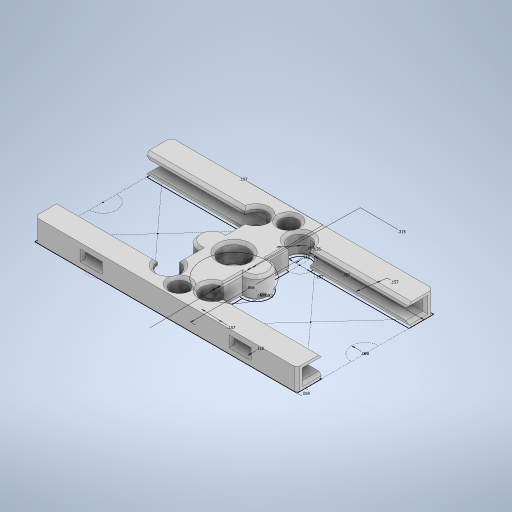
# Autodesk Inventor part: DualSensorClip-v2
Saved by Autodesk Inventor 2023 (Build 270158030, 158C)
## iProperties
Created: 2024-03-05
Part Number: DualSensorClip-v2
Material: Generic
Document SubType Name: Modeling
Designer: lvrectanus0
Density: 1 g/cm^3
Appearance: Default
Author: lvrectanus0
Autodesk Inventor part; units mm, degrees
ref_plane "YZ Plane" through (0, 0, 0) normal (1, 0, 0) x (0, 1, 0)
ref_plane "XZ Plane" through (0, 0, 0) normal (0, 1, 0) x (-1, 0, 0)
ref_plane "XY Plane" through (0, 0, 0) normal (0, 0, 1) x (1, 0, 0)
sketch "Sketch1" plane through (0, 0, 0) normal (0, 1, 0) x (-1, 0, 0)
  circle A0 centre (0, 0) radius 2.5
  circle A1 centre (0, 0) radius 4
  arc A2 (-3.21875, 2.374794) -> (-3.21875, -2.374794) centre (-4, 0) ccw
  line L0 (-24, 11) -> (-4, 11) construction
  line L1 (-4, 11) -> (-4, -11) construction
  line L2 (-4, -11) -> (-24, -11) construction
  line L3 (-24, -11) -> (-24, 11) construction
  line L4 (-24, 11) -> (-4, -11) construction
  line L5 (-4, 11) -> (-24, -11) construction
  arc A3 (-24, -2.5) -> (-24, 2.5) centre (-24, 0) ccw construction
  line L6 (-4, -8) -> (-24, -8) construction
  line L7 (-4, 8) -> (-24, 8) construction
  line L8 (-24, -11) -> (-3.228757, -11) construction
  line L9 (-3.228757, -11) -> (-3.228757, -12.5) construction
  line L10 (-3.228757, -12.5) -> (-24, -12.5)
  line L11 (-24, -12.5) -> (-24, -11)
  line L12 (-4, 11) -> (-24, 11) construction
  line L13 (-24, 11) -> (-24, 12.5)
  line L14 (-24, 12.5) -> (-4, 12.5)
  line L15 (-4, 12.5) -> (-4, 11) construction
  line L16 (-24, 8) -> (-24, 11)
  line L17 (-24, -8) -> (-24, -11)
  circle A4 centre (-4, -8) radius 2 construction
  circle A5 centre (-4, 8) radius 2 construction
  line L18 (-4, 2.5) -> (-4, 6)
  line L19 (-4, -2.5) -> (-4, -6)
  line L20 (-6, -8) -> (-24, -8)
  line L21 (-24, 8) -> (-6, 8)
  circle A6 centre (-13.614378, -11) radius 2 construction
  arc A7 (-6, -8) -> (-4, -6) centre (-4, -8) ccw
  circle A8 centre (0, -10) radius 1.6
  line L22 (-4, -10) -> (-1.6, -10) construction
  line L23 (0, -4) -> (0, -8.4) construction
  arc A9 (-4, 6) -> (-6, 8) centre (-4, 8) ccw
  arc A10 (3.21875, -2.374794) -> (3.21875, 2.374794) centre (4, 0) ccw
  line L24 (4, 2.5) -> (4, 6)
  line L25 (4, -11) -> (4, 11) construction
  circle A11 centre (13.614378, 11) radius 2 construction
  line L26 (24, -12.5) -> (4, -12.5)
  line L27 (24, -8) -> (6, -8)
  line L28 (4, -8) -> (24, -8) construction
  line L29 (4, -11) -> (24, -11) construction
  line L30 (24, -11) -> (4, -11) construction
  arc A12 (24, 2.5) -> (24, -2.5) centre (24, 0) ccw construction
  line L31 (6, 8) -> (24, 8)
  line L32 (4, 8) -> (24, 8) construction
  line L33 (3.228757, 12.5) -> (24, 12.5)
  line L34 (24, 8) -> (24, 11)
  line L35 (24, 11) -> (3.228757, 11) construction
  line L36 (4, 11) -> (24, 11) construction
  line L37 (4, -11) -> (24, 11) construction
  line L38 (24, 11) -> (24, -11) construction
  line L39 (24, -11) -> (4, 11) construction
  line L40 (4, -2.5) -> (4, -6)
  line L41 (24, 12.5) -> (24, 11)
  line L42 (3.228757, 11) -> (3.228757, 12.5) construction
  line L43 (24, -8) -> (24, -11)
  line L44 (24, -11) -> (24, -12.5)
  circle A13 centre (4, -8) radius 2 construction
  arc A14 (4, -6) -> (6, -8) centre (4, -8) ccw
  line L45 (4, -12.5) -> (4, -11) construction
  arc A15 (6, 8) -> (4, 6) centre (4, 8) ccw
  circle A16 centre (4, 8) radius 2 construction
  line L46 (0, 4) -> (0, 8.4) construction
  line L47 (4, 10) -> (1.6, 10) construction
  circle A17 centre (0, 10) radius 1.6
  line L48 (4, -12.5) -> (-3.228757, -12.5)
  line L49 (3.228757, 12.5) -> (-4, 12.5)
  point P0 (-14, 0)
  point P1 (14, 0)
  dimension "d0" = 5
  dimension "d1" = 8
  dimension "d2" = 2.5
  dimension "d3" = 22
  dimension "d4" = 20
  dimension "d5" = 2.5
  dimension "d6" = 3
  dimension "d7" = 3
  dimension "d8" = 1.5
  dimension "d9" = 1.5
  dimension "d10" = 4
  dimension "d11" = 4
  dimension "d12" = 4
  dimension "d13" = 3.2
  dimension "d16" = 360
  constraints: 96 end point, 38 point on circle, 18 centre point, 14 coincident, 12 point on line, 6 midpoint, 6 parallel, 4 horizontal, 4 perpendicular, 3 collinear, 2 horizontal alignment, 2 tangent, 1 vertical, 1 vertical alignment, 164 other
  measures "d0" diameter of A0
  measures "d1" diameter of A1
  measures "d2" radius of A2
  measures "d3" distance of L0.end L2.start
  measures "d4" distance of L2.start L2.end
  measures "d5" radius of A3
  measures "d6" distance between parallel lines of L2 L6
  measures "d7" distance between parallel lines of L7 L0
  measures "d8" distance of L8.end L9.end
  measures "d9" distance of L12.end L13.end
  measures "d10" diameter of A4
  measures "d11" diameter of A5
  measures "d12" diameter of A6
  measures "d13" diameter of A8
extrude "Extrusion1" add sketch "Sketch1" along normal blind 4
sketch "Sketch2" plane through (24, 0, 12.5) normal (1, 0, 0) x (0, 0, -1)
  line L0 (1.5, 3) -> (23.5, 3)
  line L1 (23.5, 3) -> (23.5, 1)
  line L2 (23.5, 1) -> (1.5, 1)
  line L3 (1.5, 1) -> (1.5, 3)
  line L4 (6.5, 4) -> (10, 4) projected
  line L5 (20.5, 0) -> (25, 0) projected
  line L6 (0, 0) -> (0, 4) projected
  line L7 (25, 0) -> (25, 4) projected
  line L8 (10, 0) -> (10, 4) projected
  line L9 (10, 1) -> (10, 3)
  line L10 (15, 0) -> (15, 4) projected
  line L11 (15, 3) -> (15, 1)
  point P0 (12.5, 0)
  point P1 (25, 2)
  dimension "d20" = 1
  dimension "d21" = 1
  dimension "d22" = 1.5
  dimension "d23" = 1.5
  constraints: 12 end point, 8 point on line, 2 parallel, 1 horizontal, 1 midpoint, 1 perpendicular
  measures "d20" distance between parallel lines of L4 L0
  measures "d21" distance between parallel lines of L5 L2
  measures "d22" distance between parallel lines of L6 L3
  measures "d23" distance from line of point (25, 2) L1
extrude "Extrusion2" cut sketch "Sketch2" against normal up to surface (20 mm away) contours L0 L8 L2 L3 | L0 L1 L2 L10
sketch "Sketch3" plane through (-24, 0, 8) normal (-1, 0, 0) x (0, 0, 1)
  line L0 (3, 1) -> (-19, 1)
  line L1 (-19, 1) -> (-19, 3)
  line L2 (-19, 3) -> (3, 3)
  line L3 (3, 3) -> (3, 1)
  line L4 (-20.5, 0) -> (-16, 0) projected
  line L5 (-20.5, 4) -> (-16, 4) projected
  line L6 (-20.5, 0) -> (-20.5, 4) projected
  line L7 (4.5, 0) -> (4.5, 4) projected
  line L8 (-5.5, 0) -> (-5.5, 4) projected
  line L9 (-5.5, 1) -> (-5.5, 3)
  line L10 (-10.5, 0) -> (-10.5, 4) projected
  line L11 (-10.5, 1) -> (-10.5, 3)
  point P0 (-8, 0)
  dimension "d26" = 1
  dimension "d27" = 1
  dimension "d28" = 1.5
  dimension "d29" = 1.5
  constraints: 12 end point, 8 point on line, 2 parallel, 1 horizontal, 1 perpendicular
  measures "d26" distance between parallel lines of L4 L0
  measures "d27" distance between parallel lines of L5 L2
  measures "d28" distance between parallel lines of L6 L1
  measures "d29" distance between parallel lines of L7 L3
extrude "Extrusion3" cut sketch "Sketch3" against normal up to surface (20 mm away) contours L0 L8 L2 L3 | L0 L1 L2 L10
sketch "Sketch4" plane through (24, 0, -12.5) normal (0, 0, -1) x (-1, 0, 0)
  line L0 (12.385622, 0) -> (8.385622, 0) construction
  line L1 (39.614378, 0) -> (35.614378, 0) construction
  line L2 (0, 0) -> (48, 0)
  line L3 (48, 0) -> (48, 4)
  line L4 (0, 4) -> (48, 4)
  line L5 (0, 0) -> (0, 4)
  line L6 (8.385622, 0) -> (8.385622, 4)
  line L7 (0, 0) -> (48, 0)
  line L8 (12.385622, 0) -> (12.385622, 4)
  line L9 (48, 4) -> (0, 4)
  line L10 (39.614378, 0) -> (39.614378, 4)
  line L11 (35.614378, 0) -> (35.614378, 4)
  line L12 (48, 4) -> (30, 4)
  line L13 (48, 3) -> (28, 3)
  line L14 (35.614378, 3) -> (39.614378, 3)
  line L15 (48, 1) -> (28, 1)
  line L16 (39.614378, 1) -> (35.614378, 1)
  line L17 (0, 1) -> (20, 1)
  line L18 (8.385622, 1) -> (12.385622, 1)
  line L19 (18, 3) -> (0, 3)
  line L20 (12.385622, 3) -> (8.385622, 3)
  point P0 (24, 0)
  constraints: 20 point on line, 16 end point, 3 perpendicular, 1 vertical
extrude "Extrusion4" cut sketch "Sketch4" against normal through all contours L6 L19 L8 L17 | L11 L13 L10 L15
chamfer "Chamfer1" distance 0.5 angle 45 58 edges at (15.6144, 2, -11) (11.6144, 2, -11) (-15.6144, 2, -11) (11.6144, 2, 11) (15.6144, 2, 11) (-11.6144, 2, -11) (-11.6144, 2, 11) (-15.6144, 2, 11) (15, 4, 8) (-15, 4, 8) (15, 4, -8) (-15, 4, -8) (-15, 0, 8) (15, 0, 8) (-15, 0, -8) (15, 0, -8) (-24, 2, 12.5) (-24, 2, -12.5) (24, 2, -12.5) (24, 2, 12.5) (-6.5, 4, 0) (-4, 4, -4.25) (-4, 4, 4.25) (-2.5858, 4, 9.4142) (-2.5858, 4, -9.4142) (2.5858, 4, -9.4142) (4, 4, -4.25) (6.5, 4, 0) (4, 4, 4.25) (2.5858, 4, 9.4142) (1.6, 4, 10) (1.6, 4, -10) (-2.5858, 0, -9.4142) (1.6, 0, -10) (2.5858, 0, -9.4142) (4, 0, -4.25) (-4, 0, -4.25) (-6.5, 0, 0) (6.5, 0, 0) (4, 0, 4.25) (-4, 0, 4.25) (-2.5858, 0, 9.4142) (2.5858, 0, 9.4142) (1.6, 0, 10) (2.5, 0, 0) (2.5, 4, 0) (-24, 3, -9.5) (-24, 1, -9.5) (-24, 3, 9.5) (-24, 1, 9.5) (-24, 2, 11) (-24, 2, -11) (24, 3, 9.5) (24, 2, 11) (24, 1, 9.5) (24, 3, -9.5) (24, 2, -11) (24, 1, -9.5)
body "Solid1"
